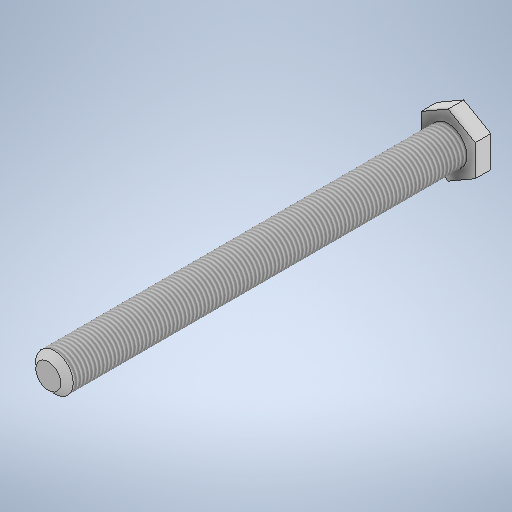
# Autodesk Inventor part: peça_002_001
Saved by Autodesk Inventor 2026 (Build 300175000, 175)
## iProperties
Created: 2025-04-08
Part Number: peça_002_001
Material: Generic
Document SubType Name: Modeling
Designer: Carlos Dias
Density: 1 g/cm^3
Appearance: Default
Author: Carlos Dias
Autodesk Inventor part; units mm, degrees
sketch "Sketch1" plane through (0, 0, 0) normal (0, 0, 1) x (1, 0, 0)
  circle A0 centre (0, 0) radius 6
  dimension "d0" = 12
  constraints: 1 centre point, 1 coincident
  measures "d0" diameter of A0
extrude "Extrusion1" add sketch "Sketch1" along normal mid plane 128
sketch "Sketch2" plane through (0, 0, -64) normal (0, 0, -1) x (-1, 0, 0)
  line L0 (0, 10) -> (8.6603, 5)
  line L1 (8.6603, 5) -> (8.6603, -5)
  line L2 (8.6603, -5) -> (0, -10)
  line L3 (0, -10) -> (-8.6603, -5)
  line L4 (-8.6603, -5) -> (-8.6603, 5)
  line L5 (-8.6603, 5) -> (0, 10)
  point P0 (0, 0)
  point P1 (0, 0)
  dimension "d3" = 10
  constraints: 12 end point, 1 coincident, 1 vertical, 13 other
  measures "d3" distance of L0.end L1.end
extrude "Extrusion2" add sketch "Sketch2" along normal blind 5
thread "Thread1" size "M12x1.25" class "6g" standard "ANSI Metric M Profile" full length
chamfer "Chamfer1" distance 2 angle 45 1 edges at (-6, 0, 64)
body "Solid1"
